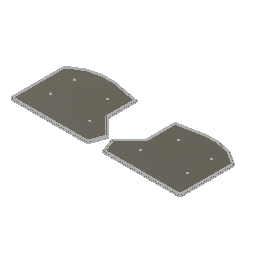
bottom (Autodesk Fusion 360 design; units mm, degrees)
Autodesk Fusion 360 part; units mm, degrees
note: some values were not read from the file. Set by a fixed rule: the direction of a hole.
sketch "case_bottom" plane through (0, 0, 0) normal (0, 0, 1) x (1, 0, 0)
  line L0 (-13.7052, -112.72) -> (-6.0652, -91.7293)
  line L1 (-111.8983, -18.5688) -> (-131.5, -30.9488)
  line L2 (-72.3112, -13.518) -> (-72.4047, -13.5)
  line L3 (-131.5, -30.9488) -> (-131.5, -112.72)
  line L4 (-32.5, -65.3353) -> (-32.5, -21.174)
  line L5 (-91.6231, -13.5) -> (-111.8983, -18.5688)
  line L6 (-72.4047, -13.5) -> (-91.6231, -13.5)
  line L7 (-131.5, -112.72) -> (-13.7052, -112.72)
  line L8 (-6.0652, -91.7293) -> (-32.5, -65.3353)
  line L9 (-32.5, -21.174) -> (-72.3112, -13.518)
  line L10 (-91.9924, -10.5) -> (-113.0931, -15.7752)
  line L11 (-134.5, -29.2953) -> (-134.5, -115.72)
  line L12 (-72.1189, -10.5) -> (-91.9924, -10.5)
  line L13 (-11.6046, -115.72) -> (-2.5919, -90.9579)
  line L14 (-134.5, -115.72) -> (-11.6046, -115.72)
  line L15 (-29.5, -18.6959) -> (-72.1189, -10.5)
  line L16 (-29.5, -64.0913) -> (-29.5, -18.6959)
  line L17 (-113.0931, -15.7752) -> (-134.5, -29.2953)
  line L18 (-2.5919, -90.9579) -> (-29.5, -64.0913)
  line L19 (-31.3, -20.1828) -> (-72.2904, -12.3)
  line L20 (-91.7708, -12.3) -> (-112.3762, -17.4513)
  line L21 (-31.3, -64.8377) -> (-31.3, -20.1828)
  line L22 (-132.7, -30.2874) -> (-132.7, -113.92)
  line L23 (-112.3762, -17.4513) -> (-132.7, -30.2874)
  line L24 (-72.2904, -12.3) -> (-91.7708, -12.3)
  line L25 (-4.6759, -91.4207) -> (-31.3, -64.8377)
  line L26 (-132.7, -113.92) -> (-12.865, -113.92)
  line L27 (-12.865, -113.92) -> (-4.6759, -91.4207)
  line L28 (-112.6152, -16.8926) -> (-133.3, -29.9567)
  line L29 (-12.4448, -114.52) -> (-3.9812, -91.2664)
  line L30 (-30.7, -19.6872) -> (-71.9712, -11.7504)
  line L31 (-3.9812, -91.2664) -> (-30.7, -64.5889)
  line L32 (-133.3, -29.9567) -> (-133.3, -114.52)
  line L33 (-91.8447, -11.7) -> (-112.6152, -16.8926)
  line L34 (-72.2332, -11.7) -> (-91.8447, -11.7)
  line L35 (-30.7, -64.5889) -> (-30.7, -19.6872)
  line L36 (-133.3, -114.52) -> (-12.4448, -114.52)
  line L37 (-71.9712, -11.7504) -> (-72.2332, -11.7)
  circle A0 centre (-108, -39.5) radius 2.2
  circle A1 centre (-108, -77.5) radius 2.2
  circle A2 centre (-56, -39.5) radius 2.2
  circle A3 centre (-39.8644, -83.3241) radius 2.2
  line L38 (-96.5, -91.61) -> (-129.5, -91.61)
  line L39 (-96.5, -109.61) -> (-96.5, -91.61)
  line L40 (-129.5, -109.61) -> (-96.5, -109.61)
  line L41 (-129.5, -91.61) -> (-129.5, -109.61)
  line L42 (-92.975, -106.99) -> (-92.975, -112.84)
  line L43 (-84.175, -112.84) -> (-84.175, -106.99)
  line L44 (-84.175, -106.99) -> (-92.975, -106.99)
  line L45 (-82.175, -107.975) -> (-82.175, -111.475)
  line L46 (-73.175, -107.975) -> (-82.175, -107.975)
  line L47 (-82.175, -111.475) -> (-73.175, -111.475)
  line L48 (-73.175, -111.475) -> (-73.175, -107.975)
  line L49 (-17.3936, -82.1718) -> (-25.1718, -74.3936)
  line L50 (-25.1718, -74.3936) -> (-31.6064, -80.8282)
  line L51 (-31.6064, -80.8282) -> (-23.8282, -88.6064)
  line L52 (-23.8282, -88.6064) -> (-17.3936, -82.1718)
  line L53 (-96.8, -79.55) -> (-105.4, -79.55)
  line L54 (-105.4, -88.45) -> (-96.8, -88.45)
  line L55 (-96.8, -88.45) -> (-96.8, -79.55)
  line L56 (-105.4, -79.55) -> (-105.4, -88.45)
extrude "Extrude1" add sketch "case_bottom" along normal blind 1.6 contours L0 L1 L2 L3 L4 L5 L6 L7 L8 L9 L42 L43 L44 | L7 L42 L43 L44 | A0 | A1 | A2 | A3 | L38 L39 L40 L41 | L45 L46 L47 L48 | L49 L50 L51 L52 | L53 L54 L55 L56 makes body 1
extrude "Extrude2" add sketch "case_bottom" along normal blind 2.8 contours L19 L20 L21 L22 L23 L24 L25 L26 L27 bodies 1
extrude "Extrude3" add sketch "case_bottom" along normal blind 1.6 contours L10 L11 L12 L13 L14 L15 L16 L17 L18 | L28 L29 L30 L31 L32 L33 L34 L35 L36 L37 bodies 1
hole "Hole1" at (-56, -39.5, 0) at (-108, -77.5, 0) at (-108, -39.5, 0) at (-39.8644, -83.3241, 0) direction (0, 0, 1) diameter 2.4 depth 1.6 tip angle 118 countersink diameter 4.4 countersink angle 90 bodies 1
fillet "Fillet1" radius 5 17 edges at (-12.865, -113.92, 2.2) (-11.6046, -115.72, 0.8) (-13.7052, -112.72, 2.2) (-134.5, -115.72, 0.8) (-132.7, -113.92, 2.2) (-131.5, -112.72, 2.2) (-131.5, -30.9488, 2.2) (-132.7, -30.2874, 2.2) (-134.5, -29.2953, 0.8) (-112.3762, -17.4513, 2.2) (-113.0931, -15.7752, 0.8) (-91.7708, -12.3, 2.2) (-91.9924, -10.5, 0.8) (-72.2904, -12.3, 2.2) (-72.1189, -10.5, 0.8) (-91.6231, -13.5, 2.2) (-111.8983, -18.5688, 2.2) on bodies 1
mirror "Mirror1" about plane through (0, 0, 0) normal (1, 0, 0) of bodies 1 makes body 2
